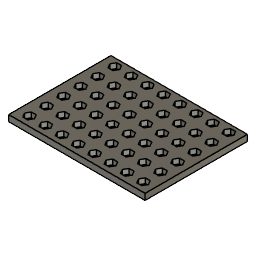
Cheesboard (Autodesk Fusion 360 design; units mm, degrees)
part number: 2025-11-09-12-34-21-661
Autodesk Fusion 360 part; units mm, degrees
(part 1 of 2)
sketch "Sketch1" plane through (0, 0, 0) normal (0, 0, 1) x (1, 0, 0)
  line L0 (0, 0) -> (176, 0)
  line L1 (176, 0) -> (176, 132)
  line L2 (176, 132) -> (0, 132)
  line L3 (0, 132) -> (0, 0)
  dimension "d1" = 132
  dimension "d2" = 176
  constraint horizontal L0
  constraint vertical L1
  constraint horizontal L2
  constraint vertical L3
  constraint coincident L0.start L3.end
  measures "d1" distance of L0.start L2.end
  measures "d2" distance of L1.end L2.end
extrude "Extrude1" add sketch "Sketch1" along normal blind 8
sketch "Sketch2" plane through (0, 0, 8) normal (0, 0, 1) x (-1, 0, 0)
  line L0 (0, -132) -> (0, 0)
  line L1 (0, 0) -> (-176, 0)
  line L2 (-176, 0) -> (-176, -132)
  line L3 (-176, -132) -> (0, -132)
  line L4 (-21.3509, -122) -> (-18.1754, -127.5)
  line L5 (-18.1754, -127.5) -> (-11.8246, -127.5)
  line L6 (-11.8246, -127.5) -> (-8.6491, -122)
  line L7 (-8.6491, -122) -> (-11.8246, -116.5)
  line L8 (-11.8246, -116.5) -> (-18.1754, -116.5)
  line L9 (-18.1754, -116.5) -> (-21.3509, -122)
  line L10 (-39.1754, -116.5) -> (-42.3509, -122)
  line L11 (-32.8246, -116.5) -> (-39.1754, -116.5)
  line L12 (-32.8246, -127.5) -> (-29.6491, -122)
  line L13 (-39.1754, -127.5) -> (-32.8246, -127.5)
  line L14 (-42.3509, -122) -> (-39.1754, -127.5)
  line L15 (-29.6491, -122) -> (-32.8246, -116.5)
  line L16 (-60.1754, -116.5) -> (-63.3509, -122)
  line L17 (-53.8246, -116.5) -> (-60.1754, -116.5)
  line L18 (-53.8246, -127.5) -> (-50.6491, -122)
  line L19 (-60.1754, -127.5) -> (-53.8246, -127.5)
  line L20 (-63.3509, -122) -> (-60.1754, -127.5)
  line L21 (-50.6491, -122) -> (-53.8246, -116.5)
  line L22 (-81.1754, -116.5) -> (-84.3509, -122)
  line L23 (-74.8246, -116.5) -> (-81.1754, -116.5)
  line L24 (-74.8246, -127.5) -> (-71.6491, -122)
  line L25 (-81.1754, -127.5) -> (-74.8246, -127.5)
  line L26 (-84.3509, -122) -> (-81.1754, -127.5)
  line L27 (-71.6491, -122) -> (-74.8246, -116.5)
  line L28 (-102.1754, -116.5) -> (-105.3509, -122)
  line L29 (-95.8246, -116.5) -> (-102.1754, -116.5)
  line L30 (-95.8246, -127.5) -> (-92.6491, -122)
  line L31 (-102.1754, -127.5) -> (-95.8246, -127.5)
  line L32 (-105.3509, -122) -> (-102.1754, -127.5)
  line L33 (-92.6491, -122) -> (-95.8246, -116.5)
  line L34 (-123.1754, -116.5) -> (-126.3509, -122)
  line L35 (-116.8246, -116.5) -> (-123.1754, -116.5)
  line L36 (-116.8246, -127.5) -> (-113.6491, -122)
  line L37 (-123.1754, -127.5) -> (-116.8246, -127.5)
  line L38 (-126.3509, -122) -> (-123.1754, -127.5)
  line L39 (-113.6491, -122) -> (-116.8246, -116.5)
  line L40 (-144.1754, -116.5) -> (-147.3509, -122)
  line L41 (-137.8246, -116.5) -> (-144.1754, -116.5)
  line L42 (-137.8246, -127.5) -> (-134.6491, -122)
  line L43 (-144.1754, -127.5) -> (-137.8246, -127.5)
  line L44 (-147.3509, -122) -> (-144.1754, -127.5)
  line L45 (-134.6491, -122) -> (-137.8246, -116.5)
  line L46 (-165.1754, -116.5) -> (-168.3509, -122)
  line L47 (-158.8246, -116.5) -> (-165.1754, -116.5)
  line L48 (-158.8246, -127.5) -> (-155.6491, -122)
  line L49 (-165.1754, -127.5) -> (-158.8246, -127.5)
  line L50 (-168.3509, -122) -> (-165.1754, -127.5)
  line L51 (-155.6491, -122) -> (-158.8246, -116.5)
  line L52 (-18.1754, -94.5) -> (-21.3509, -100)
  line L53 (-11.8246, -94.5) -> (-18.1754, -94.5)
  line L54 (-11.8246, -105.5) -> (-8.6491, -100)
  line L55 (-18.1754, -105.5) -> (-11.8246, -105.5)
  line L56 (-21.3509, -100) -> (-18.1754, -105.5)
  line L57 (-8.6491, -100) -> (-11.8246, -94.5)
  line L58 (-39.1754, -94.5) -> (-42.3509, -100)
  line L59 (-32.8246, -94.5) -> (-39.1754, -94.5)
  line L60 (-32.8246, -105.5) -> (-29.6491, -100)
  line L61 (-39.1754, -105.5) -> (-32.8246, -105.5)
  line L62 (-42.3509, -100) -> (-39.1754, -105.5)
  line L63 (-29.6491, -100) -> (-32.8246, -94.5)
  line L64 (-60.1754, -94.5) -> (-63.3509, -100)
  line L65 (-53.8246, -94.5) -> (-60.1754, -94.5)
  line L66 (-53.8246, -105.5) -> (-50.6491, -100)
  line L67 (-60.1754, -105.5) -> (-53.8246, -105.5)
  line L68 (-63.3509, -100) -> (-60.1754, -105.5)
  line L69 (-50.6491, -100) -> (-53.8246, -94.5)
  line L70 (-81.1754, -94.5) -> (-84.3509, -100)
  line L71 (-74.8246, -94.5) -> (-81.1754, -94.5)
  line L72 (-74.8246, -105.5) -> (-71.6491, -100)
  line L73 (-81.1754, -105.5) -> (-74.8246, -105.5)
  line L74 (-84.3509, -100) -> (-81.1754, -105.5)
  line L75 (-71.6491, -100) -> (-74.8246, -94.5)
  line L76 (-102.1754, -94.5) -> (-105.3509, -100)
  line L77 (-95.8246, -94.5) -> (-102.1754, -94.5)
  line L78 (-95.8246, -105.5) -> (-92.6491, -100)
  line L79 (-102.1754, -105.5) -> (-95.8246, -105.5)
  line L80 (-105.3509, -100) -> (-102.1754, -105.5)
  line L81 (-92.6491, -100) -> (-95.8246, -94.5)
  line L82 (-123.1754, -94.5) -> (-126.3509, -100)
  line L83 (-116.8246, -94.5) -> (-123.1754, -94.5)
  line L84 (-116.8246, -105.5) -> (-113.6491, -100)
  line L85 (-123.1754, -105.5) -> (-116.8246, -105.5)
  line L86 (-126.3509, -100) -> (-123.1754, -105.5)
  line L87 (-113.6491, -100) -> (-116.8246, -94.5)
  line L88 (-144.1754, -94.5) -> (-147.3509, -100)
  line L89 (-137.8246, -94.5) -> (-144.1754, -94.5)
  line L90 (-137.8246, -105.5) -> (-134.6491, -100)
  line L91 (-144.1754, -105.5) -> (-137.8246, -105.5)
  line L92 (-147.3509, -100) -> (-144.1754, -105.5)
  line L93 (-134.6491, -100) -> (-137.8246, -94.5)
  line L94 (-165.1754, -94.5) -> (-168.3509, -100)
  line L95 (-158.8246, -94.5) -> (-165.1754, -94.5)
  line L96 (-158.8246, -105.5) -> (-155.6491, -100)
  line L97 (-165.1754, -105.5) -> (-158.8246, -105.5)
  line L98 (-168.3509, -100) -> (-165.1754, -105.5)
  line L99 (-155.6491, -100) -> (-158.8246, -94.5)
  line L100 (-18.1754, -72.5) -> (-21.3509, -78)
  line L101 (-11.8246, -72.5) -> (-18.1754, -72.5)
  line L102 (-11.8246, -83.5) -> (-8.6491, -78)
  line L103 (-18.1754, -83.5) -> (-11.8246, -83.5)
  line L104 (-21.3509, -78) -> (-18.1754, -83.5)
  line L105 (-8.6491, -78) -> (-11.8246, -72.5)
  line L106 (-39.1754, -72.5) -> (-42.3509, -78)
  line L107 (-32.8246, -72.5) -> (-39.1754, -72.5)
  line L108 (-32.8246, -83.5) -> (-29.6491, -78)
  line L109 (-39.1754, -83.5) -> (-32.8246, -83.5)
  line L110 (-42.3509, -78) -> (-39.1754, -83.5)
  line L111 (-29.6491, -78) -> (-32.8246, -72.5)
  line L112 (-60.1754, -72.5) -> (-63.3509, -78)
  line L113 (-53.8246, -72.5) -> (-60.1754, -72.5)
  line L114 (-53.8246, -83.5) -> (-50.6491, -78)
  line L115 (-60.1754, -83.5) -> (-53.8246, -83.5)
  line L116 (-63.3509, -78) -> (-60.1754, -83.5)
  line L117 (-50.6491, -78) -> (-53.8246, -72.5)
  line L118 (-81.1754, -72.5) -> (-84.3509, -78)
  line L119 (-74.8246, -72.5) -> (-81.1754, -72.5)
  line L120 (-74.8246, -83.5) -> (-71.6491, -78)
  line L121 (-81.1754, -83.5) -> (-74.8246, -83.5)
  line L122 (-84.3509, -78) -> (-81.1754, -83.5)
  line L123 (-71.6491, -78) -> (-74.8246, -72.5)
  line L124 (-102.1754, -72.5) -> (-105.3509, -78)
  line L125 (-95.8246, -72.5) -> (-102.1754, -72.5)
  line L126 (-95.8246, -83.5) -> (-92.6491, -78)
  line L127 (-102.1754, -83.5) -> (-95.8246, -83.5)
  line L128 (-105.3509, -78) -> (-102.1754, -83.5)
  line L129 (-92.6491, -78) -> (-95.8246, -72.5)
  line L130 (-123.1754, -72.5) -> (-126.3509, -78)
  line L131 (-116.8246, -72.5) -> (-123.1754, -72.5)
  line L132 (-116.8246, -83.5) -> (-113.6491, -78)
  line L133 (-123.1754, -83.5) -> (-116.8246, -83.5)
  line L134 (-126.3509, -78) -> (-123.1754, -83.5)
  line L135 (-113.6491, -78) -> (-116.8246, -72.5)
  line L136 (-144.1754, -72.5) -> (-147.3509, -78)
  line L137 (-137.8246, -72.5) -> (-144.1754, -72.5)
  line L138 (-137.8246, -83.5) -> (-134.6491, -78)
  line L139 (-144.1754, -83.5) -> (-137.8246, -83.5)
  line L140 (-147.3509, -78) -> (-144.1754, -83.5)
  line L141 (-134.6491, -78) -> (-137.8246, -72.5)
  line L142 (-165.1754, -72.5) -> (-168.3509, -78)
  line L143 (-158.8246, -72.5) -> (-165.1754, -72.5)
  line L144 (-158.8246, -83.5) -> (-155.6491, -78)
  line L145 (-165.1754, -83.5) -> (-158.8246, -83.5)
  line L146 (-168.3509, -78) -> (-165.1754, -83.5)
  line L147 (-155.6491, -78) -> (-158.8246, -72.5)
  line L148 (-18.1754, -50.5) -> (-21.3509, -56)
  line L149 (-11.8246, -50.5) -> (-18.1754, -50.5)
  line L150 (-11.8246, -61.5) -> (-8.6491, -56)
  line L151 (-18.1754, -61.5) -> (-11.8246, -61.5)
  line L152 (-21.3509, -56) -> (-18.1754, -61.5)
  line L153 (-8.6491, -56) -> (-11.8246, -50.5)
  line L154 (-39.1754, -50.5) -> (-42.3509, -56)
  line L155 (-32.8246, -50.5) -> (-39.1754, -50.5)
  line L156 (-32.8246, -61.5) -> (-29.6491, -56)
  line L157 (-39.1754, -61.5) -> (-32.8246, -61.5)
  line L158 (-42.3509, -56) -> (-39.1754, -61.5)
  line L159 (-29.6491, -56) -> (-32.8246, -50.5)
  line L160 (-60.1754, -50.5) -> (-63.3509, -56)
  line L161 (-53.8246, -50.5) -> (-60.1754, -50.5)
  line L162 (-53.8246, -61.5) -> (-50.6491, -56)
  line L163 (-60.1754, -61.5) -> (-53.8246, -61.5)
  line L164 (-63.3509, -56) -> (-60.1754, -61.5)
  line L165 (-50.6491, -56) -> (-53.8246, -50.5)
  line L166 (-81.1754, -50.5) -> (-84.3509, -56)
  line L167 (-74.8246, -50.5) -> (-81.1754, -50.5)
  line L168 (-74.8246, -61.5) -> (-71.6491, -56)
  line L169 (-81.1754, -61.5) -> (-74.8246, -61.5)
  line L170 (-84.3509, -56) -> (-81.1754, -61.5)
  line L171 (-71.6491, -56) -> (-74.8246, -50.5)
  line L172 (-102.1754, -50.5) -> (-105.3509, -56)
  line L173 (-95.8246, -50.5) -> (-102.1754, -50.5)
  line L174 (-95.8246, -61.5) -> (-92.6491, -56)
  line L175 (-102.1754, -61.5) -> (-95.8246, -61.5)
  line L176 (-105.3509, -56) -> (-102.1754, -61.5)
  line L177 (-92.6491, -56) -> (-95.8246, -50.5)
  line L178 (-123.1754, -50.5) -> (-126.3509, -56)
  line L179 (-116.8246, -50.5) -> (-123.1754, -50.5)
  line L180 (-116.8246, -61.5) -> (-113.6491, -56)
  line L181 (-123.1754, -61.5) -> (-116.8246, -61.5)
  line L182 (-126.3509, -56) -> (-123.1754, -61.5)
  line L183 (-113.6491, -56) -> (-116.8246, -50.5)
  line L184 (-144.1754, -50.5) -> (-147.3509, -56)
  line L185 (-137.8246, -50.5) -> (-144.1754, -50.5)
  line L186 (-137.8246, -61.5) -> (-134.6491, -56)
  line L187 (-144.1754, -61.5) -> (-137.8246, -61.5)
  line L188 (-147.3509, -56) -> (-144.1754, -61.5)
  line L189 (-134.6491, -56) -> (-137.8246, -50.5)
  line L190 (-165.1754, -50.5) -> (-168.3509, -56)
  line L191 (-158.8246, -50.5) -> (-165.1754, -50.5)
  line L192 (-158.8246, -61.5) -> (-155.6491, -56)
  line L193 (-165.1754, -61.5) -> (-158.8246, -61.5)
  line L194 (-168.3509, -56) -> (-165.1754, -61.5)
  line L195 (-155.6491, -56) -> (-158.8246, -50.5)
  line L196 (-18.1754, -28.5) -> (-21.3509, -34)
  line L197 (-11.8246, -28.5) -> (-18.1754, -28.5)
  line L198 (-11.8246, -39.5) -> (-8.6491, -34)
  line L199 (-18.1754, -39.5) -> (-11.8246, -39.5)
  line L200 (-21.3509, -34) -> (-18.1754, -39.5)
  line L201 (-8.6491, -34) -> (-11.8246, -28.5)
  line L202 (-39.1754, -28.5) -> (-42.3509, -34)
  line L203 (-32.8246, -28.5) -> (-39.1754, -28.5)
  line L204 (-32.8246, -39.5) -> (-29.6491, -34)
  line L205 (-39.1754, -39.5) -> (-32.8246, -39.5)
  line L206 (-42.3509, -34) -> (-39.1754, -39.5)
  line L207 (-29.6491, -34) -> (-32.8246, -28.5)
  line L208 (-60.1754, -28.5) -> (-63.3509, -34)
  line L209 (-53.8246, -28.5) -> (-60.1754, -28.5)
  line L210 (-53.8246, -39.5) -> (-50.6491, -34)
  line L211 (-60.1754, -39.5) -> (-53.8246, -39.5)
  line L212 (-63.3509, -34) -> (-60.1754, -39.5)
  line L213 (-50.6491, -34) -> (-53.8246, -28.5)
  line L214 (-81.1754, -28.5) -> (-84.3509, -34)
  line L215 (-74.8246, -28.5) -> (-81.1754, -28.5)
  line L216 (-74.8246, -39.5) -> (-71.6491, -34)
  line L217 (-81.1754, -39.5) -> (-74.8246, -39.5)
  line L218 (-84.3509, -34) -> (-81.1754, -39.5)
  line L219 (-71.6491, -34) -> (-74.8246, -28.5)
  line L220 (-102.1754, -28.5) -> (-105.3509, -34)
  line L221 (-95.8246, -28.5) -> (-102.1754, -28.5)
  line L222 (-95.8246, -39.5) -> (-92.6491, -34)
  line L223 (-102.1754, -39.5) -> (-95.8246, -39.5)
  line L224 (-105.3509, -34) -> (-102.1754, -39.5)
  line L225 (-92.6491, -34) -> (-95.8246, -28.5)
  line L226 (-123.1754, -28.5) -> (-126.3509, -34)
  line L227 (-116.8246, -28.5) -> (-123.1754, -28.5)
  line L228 (-116.8246, -39.5) -> (-113.6491, -34)
  line L229 (-123.1754, -39.5) -> (-116.8246, -39.5)
  line L230 (-126.3509, -34) -> (-123.1754, -39.5)
  line L231 (-113.6491, -34) -> (-116.8246, -28.5)
  line L232 (-144.1754, -28.5) -> (-147.3509, -34)
  line L233 (-137.8246, -28.5) -> (-144.1754, -28.5)
  line L234 (-137.8246, -39.5) -> (-134.6491, -34)
  line L235 (-144.1754, -39.5) -> (-137.8246, -39.5)
  line L236 (-147.3509, -34) -> (-144.1754, -39.5)
  line L237 (-134.6491, -34) -> (-137.8246, -28.5)
  line L238 (-165.1754, -28.5) -> (-168.3509, -34)
  line L239 (-158.8246, -28.5) -> (-165.1754, -28.5)
  line L240 (-158.8246, -39.5) -> (-155.6491, -34)
  line L241 (-165.1754, -39.5) -> (-158.8246, -39.5)
  line L242 (-168.3509, -34) -> (-165.1754, -39.5)
  line L243 (-155.6491, -34) -> (-158.8246, -28.5)
  line L244 (-18.1754, -6.5) -> (-21.3509, -12)
  line L245 (-11.8246, -6.5) -> (-18.1754, -6.5)
  line L246 (-11.8246, -17.5) -> (-8.6491, -12)
  line L247 (-18.1754, -17.5) -> (-11.8246, -17.5)
  line L248 (-21.3509, -12) -> (-18.1754, -17.5)
  line L249 (-8.6491, -12) -> (-11.8246, -6.5)
  line L250 (-39.1754, -6.5) -> (-42.3509, -12)
  line L251 (-32.8246, -6.5) -> (-39.1754, -6.5)
  line L252 (-32.8246, -17.5) -> (-29.6491, -12)
  line L253 (-39.1754, -17.5) -> (-32.8246, -17.5)
  line L254 (-42.3509, -12) -> (-39.1754, -17.5)
  line L255 (-29.6491, -12) -> (-32.8246, -6.5)
  line L256 (-60.1754, -6.5) -> (-63.3509, -12)
  line L257 (-53.8246, -6.5) -> (-60.1754, -6.5)
  line L258 (-53.8246, -17.5) -> (-50.6491, -12)
  line L259 (-60.1754, -17.5) -> (-53.8246, -17.5)
  line L260 (-63.3509, -12) -> (-60.1754, -17.5)
  line L261 (-50.6491, -12) -> (-53.8246, -6.5)
  line L262 (-81.1754, -6.5) -> (-84.3509, -12)
  line L263 (-74.8246, -6.5) -> (-81.1754, -6.5)
  line L264 (-74.8246, -17.5) -> (-71.6491, -12)
  line L265 (-81.1754, -17.5) -> (-74.8246, -17.5)
  line L266 (-84.3509, -12) -> (-81.1754, -17.5)
  line L267 (-71.6491, -12) -> (-74.8246, -6.5)
  line L268 (-102.1754, -6.5) -> (-105.3509, -12)
  line L269 (-95.8246, -6.5) -> (-102.1754, -6.5)
  line L270 (-95.8246, -17.5) -> (-92.6491, -12)
  line L271 (-102.1754, -17.5) -> (-95.8246, -17.5)
  line L272 (-105.3509, -12) -> (-102.1754, -17.5)
  line L273 (-92.6491, -12) -> (-95.8246, -6.5)
  line L274 (-123.1754, -6.5) -> (-126.3509, -12)
  line L275 (-116.8246, -6.5) -> (-123.1754, -6.5)
  line L276 (-116.8246, -17.5) -> (-113.6491, -12)
  line L277 (-123.1754, -17.5) -> (-116.8246, -17.5)
  line L278 (-126.3509, -12) -> (-123.1754, -17.5)
  line L279 (-113.6491, -12) -> (-116.8246, -6.5)
  line L280 (-144.1754, -6.5) -> (-147.3509, -12)
  line L281 (-137.8246, -6.5) -> (-144.1754, -6.5)
  line L282 (-137.8246, -17.5) -> (-134.6491, -12)
  line L283 (-144.1754, -17.5) -> (-137.8246, -17.5)
  line L284 (-147.3509, -12) -> (-144.1754, -17.5)
  line L285 (-134.6491, -12) -> (-137.8246, -6.5)
  line L286 (-165.1754, -6.5) -> (-168.3509, -12)
  line L287 (-158.8246, -6.5) -> (-165.1754, -6.5)
  line L288 (-158.8246, -17.5) -> (-155.6491, -12)
  line L289 (-165.1754, -17.5) -> (-158.8246, -17.5)
  line L290 (-168.3509, -12) -> (-165.1754, -17.5)
  line L291 (-155.6491, -12) -> (-158.8246, -6.5)
  point P0 (-15, -122)
  point P1 (-36, -122)
  point P2 (-57, -122)
  point P3 (-78, -122)
  point P4 (-99, -122)
  point P5 (-120, -122)
  point P6 (-141, -122)
  point P7 (-162, -122)
  point P8 (-15, -100)
  point P9 (-36, -100)
  point P10 (-57, -100)
  point P11 (-78, -100)
  point P12 (-99, -100)
  point P13 (-120, -100)
  point P14 (-141, -100)
  point P15 (-162, -100)
  point P16 (-15, -78)
  point P17 (-36, -78)
  point P18 (-57, -78)
  point P19 (-78, -78)
  point P20 (-99, -78)
  point P21 (-120, -78)
  point P22 (-141, -78)
  point P23 (-162, -78)
  point P24 (-15, -56)
  point P25 (-36, -56)
  point P26 (-57, -56)
  point P27 (-78, -56)
  point P28 (-99, -56)
  point P29 (-120, -56)
  point P30 (-141, -56)
  point P31 (-162, -56)
  point P32 (-15, -34)
  point P33 (-36, -34)
  point P34 (-57, -34)
  point P35 (-78, -34)
  point P36 (-99, -34)
  point P37 (-120, -34)
  point P38 (-141, -34)
  point P39 (-162, -34)
  point P40 (-15, -12)
  point P41 (-36, -12)
  point P42 (-57, -12)
  point P43 (-78, -12)
  point P44 (-99, -12)
  point P45 (-120, -12)
  point P46 (-141, -12)
  point P47 (-162, -12)
  dimension "d6" = 11
  dimension "d7" = 10
  dimension "d8" = 15
  dimension "d11" = -21
  dimension "d12" = 22
  constraint parallel L3 L5
  measures "d6" distance of L4 L7
  measures "d7" distance of L3 P0
  measures "d8" distance of L0 P0
extrude "Extrude2" cut sketch "Sketch2" against normal blind 6.5 contours L4 L5 L6 L7 L8 L9 | L10 L11 L12 L13 L14 L15 | L16 L17 L18 L19 L20 L21 | L22 L23 L24 L25 L26 L27 | L28 L29 L30 L31 L32 L33 | L34 L35 L36 L37 L38 L39 | L40 L41 L42 L43 L44 L45 | L46 L47 L48 L49 L50 L51 | L52 L53 L54 L55 L56 L57 | L58 L59 L60 L61 L62 L63 | L64 L65 L66 L67 L68 L69 | L70 L71 L72 L73 L74 L75 | L76 L77 L78 L79 L80 L81 | L82 L83 L84 L85 L86 L87 | L88 L89 L90 L91 L92 L93 | L94 L95 L96 L97 L98 L99 | L100 L101 L102 L103 L104 L105 | L106 L107 L108 L109 L110 L111 | L112 L113 L114 L115 L116 L117 | L118 L119 L120 L121 L122 L123 | L124 L125 L126 L127 L128 L129 | L130 L131 L132 L133 L134 L135 | L136 L137 L138 L139 L140 L141 | L142 L143 L144 L145 L146 L147 | L148 L149 L150 L151 L152 L153 | L154 L155 L156 L157 L158 L159 | L160 L161 L162 L163 L164 L165 | L166 L167 L168 L169 L170 L171 | L172 L173 L174 L175 L176 L177 | L178 L179 L180 L181 L182 L183 | L184 L185 L186 L187 L188 L189 | L190 L191 L192 L193 L194 L195 | L196 L197 L198 L199 L200 L201 | L202 L203 L204 L205 L206 L207 | L208 L209 L210 L211 L212 L213 | L214 L215 L216 L217 L218 L219 | L220 L221 L222 L223 L224 L225 | L226 L227 L228 L229 L230 L231 | L232 L233 L234 L235 L236 L237 | L238 L239 L240 L241 L242 L243 | L244 L245 L246 L247 L248 L249 | L250 L251 L252 L253 L254 L255 | L256 L257 L258 L259 L260 L261 | L262 L263 L264 L265 L266 L267 | L268 L269 L270 L271 L272 L273 | L274 L275 L276 L277 L278 L279 | L280 L281 L282 L283 L284 L285 | L286 L287 L288 L289 L290 L291
sketch "Sketch3" plane through (0, 0, 8) normal (0, 0, 1) x (-1, 0, 0)
  line L0 (-123.1754, -6.5) -> (-116.8246, -6.5)
  line L1 (-116.8246, -6.5) -> (-113.6491, -12)
  line L2 (-113.6491, -12) -> (-116.8246, -17.5)
  line L3 (-116.8246, -17.5) -> (-123.1754, -17.5)
  line L4 (-123.1754, -17.5) -> (-126.3509, -12)
  line L5 (-126.3509, -12) -> (-123.1754, -6.5)
  line L6 (-39.1754, -6.5) -> (-32.8246, -6.5)
  line L7 (-32.8246, -6.5) -> (-29.6491, -12)
  line L8 (-29.6491, -12) -> (-32.8246, -17.5)
  line L9 (-32.8246, -17.5) -> (-39.1754, -17.5)
  line L10 (-39.1754, -17.5) -> (-42.3509, -12)
  line L11 (-42.3509, -12) -> (-39.1754, -6.5)
  line L12 (-123.1754, -28.5) -> (-116.8246, -28.5)
  line L13 (-116.8246, -28.5) -> (-113.6491, -34)
  line L14 (-113.6491, -34) -> (-116.8246, -39.5)
  line L15 (-116.8246, -39.5) -> (-123.1754, -39.5)
  line L16 (-123.1754, -39.5) -> (-126.3509, -34)
  line L17 (-126.3509, -34) -> (-123.1754, -28.5)
  line L18 (-39.1754, -28.5) -> (-32.8246, -28.5)
  line L19 (-32.8246, -28.5) -> (-29.6491, -34)
  line L20 (-29.6491, -34) -> (-32.8246, -39.5)
  line L21 (-32.8246, -39.5) -> (-39.1754, -39.5)
  line L22 (-39.1754, -39.5) -> (-42.3509, -34)
  line L23 (-42.3509, -34) -> (-39.1754, -28.5)
  line L24 (-123.1754, -50.5) -> (-116.8246, -50.5)
  line L25 (-116.8246, -50.5) -> (-113.6491, -56)
  line L26 (-113.6491, -56) -> (-116.8246, -61.5)
  line L27 (-116.8246, -61.5) -> (-123.1754, -61.5)
  line L28 (-123.1754, -61.5) -> (-126.3509, -56)
  line L29 (-126.3509, -56) -> (-123.1754, -50.5)
  line L30 (-39.1754, -50.5) -> (-32.8246, -50.5)
  line L31 (-32.8246, -50.5) -> (-29.6491, -56)
  line L32 (-29.6491, -56) -> (-32.8246, -61.5)
  line L33 (-32.8246, -61.5) -> (-39.1754, -61.5)
  line L34 (-39.1754, -61.5) -> (-42.3509, -56)
  line L35 (-42.3509, -56) -> (-39.1754, -50.5)
  line L36 (-123.1754, -72.5) -> (-116.8246, -72.5)
  line L37 (-116.8246, -72.5) -> (-113.6491, -78)
  line L38 (-113.6491, -78) -> (-116.8246, -83.5)
  line L39 (-116.8246, -83.5) -> (-123.1754, -83.5)
  line L40 (-123.1754, -83.5) -> (-126.3509, -78)
  line L41 (-126.3509, -78) -> (-123.1754, -72.5)
  line L42 (-39.1754, -72.5) -> (-32.8246, -72.5)
  line L43 (-32.8246, -72.5) -> (-29.6491, -78)
  line L44 (-29.6491, -78) -> (-32.8246, -83.5)
  line L45 (-32.8246, -83.5) -> (-39.1754, -83.5)
  line L46 (-39.1754, -83.5) -> (-42.3509, -78)
  line L47 (-42.3509, -78) -> (-39.1754, -72.5)
  line L48 (-123.1754, -94.5) -> (-116.8246, -94.5)
  line L49 (-116.8246, -94.5) -> (-113.6491, -100)
  line L50 (-113.6491, -100) -> (-116.8246, -105.5)
  line L51 (-116.8246, -105.5) -> (-123.1754, -105.5)
  line L52 (-123.1754, -105.5) -> (-126.3509, -100)
  line L53 (-126.3509, -100) -> (-123.1754, -94.5)
  line L54 (-39.1754, -94.5) -> (-32.8246, -94.5)
  line L55 (-32.8246, -94.5) -> (-29.6491, -100)
  line L56 (-29.6491, -100) -> (-32.8246, -105.5)
  line L57 (-32.8246, -105.5) -> (-39.1754, -105.5)
  line L58 (-39.1754, -105.5) -> (-42.3509, -100)
  line L59 (-42.3509, -100) -> (-39.1754, -94.5)
  line L60 (-123.1754, -116.5) -> (-116.8246, -116.5)
  line L61 (-116.8246, -116.5) -> (-113.6491, -122)
  line L62 (-113.6491, -122) -> (-116.8246, -127.5)
  line L63 (-116.8246, -127.5) -> (-123.1754, -127.5)
  line L64 (-123.1754, -127.5) -> (-126.3509, -122)
  line L65 (-126.3509, -122) -> (-123.1754, -116.5)
  line L66 (-18.1754, -127.5) -> (-21.3509, -122)
  line L67 (-21.3509, -122) -> (-18.1754, -116.5)
  line L68 (-18.1754, -116.5) -> (-11.8246, -116.5)
  line L69 (-11.8246, -116.5) -> (-8.6491, -122)
  line L70 (-8.6491, -122) -> (-11.8246, -127.5)
  line L71 (-11.8246, -127.5) -> (-18.1754, -127.5)
  line L72 (-60.1754, -116.5) -> (-53.8246, -116.5)
  line L73 (-53.8246, -116.5) -> (-50.6491, -122)
  line L74 (-50.6491, -122) -> (-53.8246, -127.5)
  line L75 (-53.8246, -127.5) -> (-60.1754, -127.5)
  line L76 (-60.1754, -127.5) -> (-63.3509, -122)
  line L77 (-63.3509, -122) -> (-60.1754, -116.5)
  line L78 (-144.1754, -116.5) -> (-137.8246, -116.5)
  line L79 (-137.8246, -116.5) -> (-134.6491, -122)
  line L80 (-134.6491, -122) -> (-137.8246, -127.5)
  line L81 (-137.8246, -127.5) -> (-144.1754, -127.5)
  line L82 (-144.1754, -127.5) -> (-147.3509, -122)
  line L83 (-147.3509, -122) -> (-144.1754, -116.5)
  line L84 (-60.1754, -94.5) -> (-53.8246, -94.5)
  line L85 (-53.8246, -94.5) -> (-50.6491, -100)
  line L86 (-50.6491, -100) -> (-53.8246, -105.5)
  line L87 (-53.8246, -105.5) -> (-60.1754, -105.5)
  line L88 (-60.1754, -105.5) -> (-63.3509, -100)
  line L89 (-63.3509, -100) -> (-60.1754, -94.5)
  line L90 (-144.1754, -94.5) -> (-137.8246, -94.5)
  line L91 (-137.8246, -94.5) -> (-134.6491, -100)
  line L92 (-134.6491, -100) -> (-137.8246, -105.5)
  line L93 (-137.8246, -105.5) -> (-144.1754, -105.5)
  line L94 (-144.1754, -105.5) -> (-147.3509, -100)
  line L95 (-147.3509, -100) -> (-144.1754, -94.5)
  line L96 (-60.1754, -72.5) -> (-53.8246, -72.5)
  line L97 (-53.8246, -72.5) -> (-50.6491, -78)
  line L98 (-50.6491, -78) -> (-53.8246, -83.5)
  line L99 (-53.8246, -83.5) -> (-60.1754, -83.5)
  line L100 (-60.1754, -83.5) -> (-63.3509, -78)
  line L101 (-63.3509, -78) -> (-60.1754, -72.5)
  line L102 (-144.1754, -72.5) -> (-137.8246, -72.5)
  line L103 (-137.8246, -72.5) -> (-134.6491, -78)
  line L104 (-134.6491, -78) -> (-137.8246, -83.5)
  line L105 (-137.8246, -83.5) -> (-144.1754, -83.5)
  line L106 (-144.1754, -83.5) -> (-147.3509, -78)
  line L107 (-147.3509, -78) -> (-144.1754, -72.5)
  line L108 (-60.1754, -50.5) -> (-53.8246, -50.5)
  line L109 (-53.8246, -50.5) -> (-50.6491, -56)
  line L110 (-50.6491, -56) -> (-53.8246, -61.5)
  line L111 (-53.8246, -61.5) -> (-60.1754, -61.5)
  line L112 (-60.1754, -61.5) -> (-63.3509, -56)
  line L113 (-63.3509, -56) -> (-60.1754, -50.5)
  line L114 (-144.1754, -50.5) -> (-137.8246, -50.5)
  line L115 (-137.8246, -50.5) -> (-134.6491, -56)
  line L116 (-134.6491, -56) -> (-137.8246, -61.5)
  line L117 (-137.8246, -61.5) -> (-144.1754, -61.5)
  line L118 (-144.1754, -61.5) -> (-147.3509, -56)
  line L119 (-147.3509, -56) -> (-144.1754, -50.5)
  line L120 (-60.1754, -28.5) -> (-53.8246, -28.5)
  line L121 (-53.8246, -28.5) -> (-50.6491, -34)
  line L122 (-50.6491, -34) -> (-53.8246, -39.5)
  line L123 (-53.8246, -39.5) -> (-60.1754, -39.5)
  line L124 (-60.1754, -39.5) -> (-63.3509, -34)
  line L125 (-63.3509, -34) -> (-60.1754, -28.5)
  line L126 (-144.1754, -28.5) -> (-137.8246, -28.5)
  line L127 (-137.8246, -28.5) -> (-134.6491, -34)
  line L128 (-134.6491, -34) -> (-137.8246, -39.5)
  line L129 (-137.8246, -39.5) -> (-144.1754, -39.5)
  line L130 (-144.1754, -39.5) -> (-147.3509, -34)
  line L131 (-147.3509, -34) -> (-144.1754, -28.5)
  line L132 (-60.1754, -6.5) -> (-53.8246, -6.5)
  line L133 (-53.8246, -6.5) -> (-50.6491, -12)
  line L134 (-50.6491, -12) -> (-53.8246, -17.5)
  line L135 (-53.8246, -17.5) -> (-60.1754, -17.5)
  line L136 (-60.1754, -17.5) -> (-63.3509, -12)
  line L137 (-63.3509, -12) -> (-60.1754, -6.5)
  line L138 (-144.1754, -6.5) -> (-137.8246, -6.5)
  line L139 (-137.8246, -6.5) -> (-134.6491, -12)
  line L140 (-134.6491, -12) -> (-137.8246, -17.5)
  line L141 (-137.8246, -17.5) -> (-144.1754, -17.5)
  line L142 (-144.1754, -17.5) -> (-147.3509, -12)
  line L143 (-147.3509, -12) -> (-144.1754, -6.5)
  line L144 (-102.1754, -6.5) -> (-95.8246, -6.5)
  line L145 (-95.8246, -6.5) -> (-92.6491, -12)
  line L146 (-92.6491, -12) -> (-95.8246, -17.5)
  line L147 (-95.8246, -17.5) -> (-102.1754, -17.5)
  line L148 (-102.1754, -17.5) -> (-105.3509, -12)
  line L149 (-105.3509, -12) -> (-102.1754, -6.5)
  line L150 (-18.1754, -6.5) -> (-11.8246, -6.5)
  line L151 (-11.8246, -6.5) -> (-8.6491, -12)
  line L152 (-8.6491, -12) -> (-11.8246, -17.5)
  line L153 (-11.8246, -17.5) -> (-18.1754, -17.5)
  line L154 (-18.1754, -17.5) -> (-21.3509, -12)
  line L155 (-21.3509, -12) -> (-18.1754, -6.5)
  line L156 (-102.1754, -28.5) -> (-95.8246, -28.5)
  line L157 (-95.8246, -28.5) -> (-92.6491, -34)
  line L158 (-92.6491, -34) -> (-95.8246, -39.5)
  line L159 (-95.8246, -39.5) -> (-102.1754, -39.5)
  line L160 (-102.1754, -39.5) -> (-105.3509, -34)
  line L161 (-105.3509, -34) -> (-102.1754, -28.5)
  line L162 (-18.1754, -28.5) -> (-11.8246, -28.5)
  line L163 (-11.8246, -28.5) -> (-8.6491, -34)
  line L164 (-8.6491, -34) -> (-11.8246, -39.5)
  line L165 (-11.8246, -39.5) -> (-18.1754, -39.5)
  line L166 (-18.1754, -39.5) -> (-21.3509, -34)
  line L167 (-21.3509, -34) -> (-18.1754, -28.5)
  line L168 (-102.1754, -50.5) -> (-95.8246, -50.5)
  line L169 (-95.8246, -50.5) -> (-92.6491, -56)
  line L170 (-92.6491, -56) -> (-95.8246, -61.5)
  line L171 (-95.8246, -61.5) -> (-102.1754, -61.5)
  line L172 (-102.1754, -61.5) -> (-105.3509, -56)
  line L173 (-105.3509, -56) -> (-102.1754, -50.5)
  line L174 (-18.1754, -50.5) -> (-11.8246, -50.5)
  line L175 (-11.8246, -50.5) -> (-8.6491, -56)
  line L176 (-8.6491, -56) -> (-11.8246, -61.5)
  line L177 (-11.8246, -61.5) -> (-18.1754, -61.5)
  line L178 (-18.1754, -61.5) -> (-21.3509, -56)
  line L179 (-21.3509, -56) -> (-18.1754, -50.5)
  line L180 (-102.1754, -72.5) -> (-95.8246, -72.5)
  line L181 (-95.8246, -72.5) -> (-92.6491, -78)
  line L182 (-92.6491, -78) -> (-95.8246, -83.5)
  line L183 (-95.8246, -83.5) -> (-102.1754, -83.5)
  line L184 (-102.1754, -83.5) -> (-105.3509, -78)
  line L185 (-105.3509, -78) -> (-102.1754, -72.5)
  line L186 (-18.1754, -72.5) -> (-11.8246, -72.5)
  line L187 (-11.8246, -72.5) -> (-8.6491, -78)
  line L188 (-8.6491, -78) -> (-11.8246, -83.5)
  line L189 (-11.8246, -83.5) -> (-18.1754, -83.5)
  line L190 (-18.1754, -83.5) -> (-21.3509, -78)
  line L191 (-21.3509, -78) -> (-18.1754, -72.5)
  line L192 (-102.1754, -94.5) -> (-95.8246, -94.5)
  line L193 (-95.8246, -94.5) -> (-92.6491, -100)
  line L194 (-92.6491, -100) -> (-95.8246, -105.5)
  line L195 (-95.8246, -105.5) -> (-102.1754, -105.5)
  line L196 (-102.1754, -105.5) -> (-105.3509, -100)
  line L197 (-105.3509, -100) -> (-102.1754, -94.5)
  line L198 (-18.1754, -94.5) -> (-11.8246, -94.5)
  line L199 (-11.8246, -94.5) -> (-8.6491, -100)
  line L200 (-8.6491, -100) -> (-11.8246, -105.5)
  line L201 (-11.8246, -105.5) -> (-18.1754, -105.5)
  line L202 (-18.1754, -105.5) -> (-21.3509, -100)
  line L203 (-21.3509, -100) -> (-18.1754, -94.5)
  line L204 (-102.1754, -116.5) -> (-95.8246, -116.5)
  line L205 (-95.8246, -116.5) -> (-92.6491, -122)
  line L206 (-92.6491, -122) -> (-95.8246, -127.5)
  line L207 (-95.8246, -127.5) -> (-102.1754, -127.5)
  line L208 (-102.1754, -127.5) -> (-105.3509, -122)
  line L209 (-105.3509, -122) -> (-102.1754, -116.5)
  line L210 (-39.1754, -116.5) -> (-32.8246, -116.5)
  line L211 (-32.8246, -116.5) -> (-29.6491, -122)
  line L212 (-29.6491, -122) -> (-32.8246, -127.5)
  line L213 (-32.8246, -127.5) -> (-39.1754, -127.5)
  line L214 (-39.1754, -127.5) -> (-42.3509, -122)
  line L215 (-42.3509, -122) -> (-39.1754, -116.5)
  line L216 (-81.1754, -116.5) -> (-74.8246, -116.5)
  line L217 (-74.8246, -116.5) -> (-71.6491, -122)
  line L218 (-71.6491, -122) -> (-74.8246, -127.5)
  line L219 (-74.8246, -127.5) -> (-81.1754, -127.5)
  line L220 (-81.1754, -127.5) -> (-84.3509, -122)
  line L221 (-84.3509, -122) -> (-81.1754, -116.5)
  line L222 (-165.1754, -116.5) -> (-158.8246, -116.5)
  line L223 (-158.8246, -116.5) -> (-155.6491, -122)
  line L224 (-155.6491, -122) -> (-158.8246, -127.5)
  line L225 (-158.8246, -127.5) -> (-165.1754, -127.5)
  line L226 (-165.1754, -127.5) -> (-168.3509, -122)
  line L227 (-168.3509, -122) -> (-165.1754, -116.5)
  line L228 (-81.1754, -94.5) -> (-74.8246, -94.5)
  line L229 (-74.8246, -94.5) -> (-71.6491, -100)
  line L230 (-71.6491, -100) -> (-74.8246, -105.5)
  line L231 (-74.8246, -105.5) -> (-81.1754, -105.5)
  line L232 (-81.1754, -105.5) -> (-84.3509, -100)
  line L233 (-84.3509, -100) -> (-81.1754, -94.5)
  line L234 (-165.1754, -94.5) -> (-158.8246, -94.5)
  line L235 (-158.8246, -94.5) -> (-155.6491, -100)
  line L236 (-155.6491, -100) -> (-158.8246, -105.5)
  line L237 (-158.8246, -105.5) -> (-165.1754, -105.5)
  line L238 (-165.1754, -105.5) -> (-168.3509, -100)
  line L239 (-168.3509, -100) -> (-165.1754, -94.5)
  line L240 (-81.1754, -72.5) -> (-74.8246, -72.5)
  line L241 (-74.8246, -72.5) -> (-71.6491, -78)
  line L242 (-71.6491, -78) -> (-74.8246, -83.5)
  line L243 (-74.8246, -83.5) -> (-81.1754, -83.5)
  line L244 (-81.1754, -83.5) -> (-84.3509, -78)
  line L245 (-84.3509, -78) -> (-81.1754, -72.5)
  line L246 (-165.1754, -72.5) -> (-158.8246, -72.5)
  line L247 (-158.8246, -72.5) -> (-155.6491, -78)
  line L248 (-155.6491, -78) -> (-158.8246, -83.5)
  line L249 (-158.8246, -83.5) -> (-165.1754, -83.5)
  line L250 (-165.1754, -83.5) -> (-168.3509, -78)
  line L251 (-168.3509, -78) -> (-165.1754, -72.5)
  line L252 (-81.1754, -50.5) -> (-74.8246, -50.5)
  line L253 (-74.8246, -50.5) -> (-71.6491, -56)
  line L254 (-71.6491, -56) -> (-74.8246, -61.5)
  line L255 (-74.8246, -61.5) -> (-81.1754, -61.5)
  line L256 (-81.1754, -61.5) -> (-84.3509, -56)
  line L257 (-84.3509, -56) -> (-81.1754, -50.5)
  line L258 (-165.1754, -50.5) -> (-158.8246, -50.5)
  line L259 (-158.8246, -50.5) -> (-155.6491, -56)
  line L260 (-155.6491, -56) -> (-158.8246, -61.5)
  line L261 (-158.8246, -61.5) -> (-165.1754, -61.5)
  line L262 (-165.1754, -61.5) -> (-168.3509, -56)
  line L263 (-168.3509, -56) -> (-165.1754, -50.5)
  line L264 (-81.1754, -28.5) -> (-74.8246, -28.5)
  line L265 (-74.8246, -28.5) -> (-71.6491, -34)
  line L266 (-71.6491, -34) -> (-74.8246, -39.5)
  line L267 (-74.8246, -39.5) -> (-81.1754, -39.5)
  line L268 (-81.1754, -39.5) -> (-84.3509, -34)
  line L269 (-84.3509, -34) -> (-81.1754, -28.5)
  line L270 (-165.1754, -28.5) -> (-158.8246, -28.5)
  line L271 (-158.8246, -28.5) -> (-155.6491, -34)
  line L272 (-155.6491, -34) -> (-158.8246, -39.5)
  line L273 (-158.8246, -39.5) -> (-165.1754, -39.5)
  line L274 (-165.1754, -39.5) -> (-168.3509, -34)
  line L275 (-168.3509, -34) -> (-165.1754, -28.5)
  line L276 (-81.1754, -6.5) -> (-74.8246, -6.5)
  line L277 (-74.8246, -6.5) -> (-71.6491, -12)
  line L278 (-71.6491, -12) -> (-74.8246, -17.5)
  line L279 (-74.8246, -17.5) -> (-81.1754, -17.5)
  line L280 (-81.1754, -17.5) -> (-84.3509, -12)
  line L281 (-84.3509, -12) -> (-81.1754, -6.5)
  line L282 (-165.1754, -6.5) -> (-158.8246, -6.5)
  line L283 (-158.8246, -6.5) -> (-155.6491, -12)
  line L284 (-155.6491, -12) -> (-158.8246, -17.5)
  line L285 (-158.8246, -17.5) -> (-165.1754, -17.5)
  line L286 (-165.1754, -17.5) -> (-168.3509, -12)
  line L287 (-168.3509, -12) -> (-165.1754, -6.5)
  line L288 (0, -132) -> (0, 0)
  line L289 (0, 0) -> (-176, 0)
  line L290 (-176, 0) -> (-176, -132)
  line L291 (-176, -132) -> (0, -132)
  circle A0 centre (-15, -122) radius 2.875
  line L292 (-15, -127.5) -> (-15, -116.5) construction
  line L293 (-8.6491, -122) -> (-21.3509, -122) construction
  dimension "d15" = 5.75
  constraint midpoint L71 L292.start
  constraint midpoint L68 L292.end
  constraint coincident L69.end L70.start
  constraint coincident L66.end L67.start
  constraint coincident A0.centre L292
  constraint coincident A0.centre L293
  measures "d15" diameter of A0
extrude "Extrude3" cut sketch "Sketch3" against normal up to surface (8 mm away) contours A0